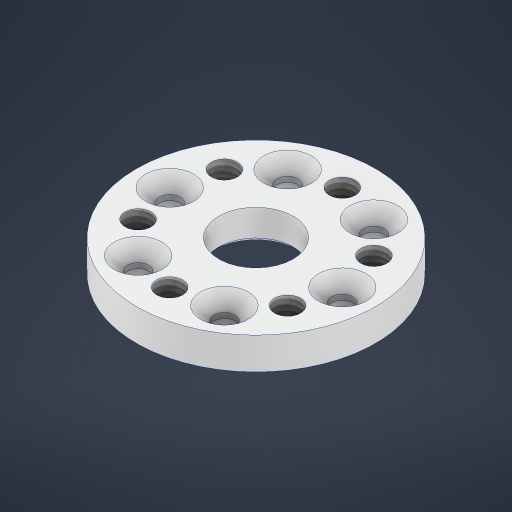
# Autodesk Inventor part: Carier_Plate_GB
Saved by Autodesk Inventor 2024.2 (Build 282272000, 272)
## iProperties
Created: 2026-01-04
Part Number: Carier_Plate_GB
Material: Aluminum 6061
Document SubType Name: Modeling
Designer: 4aida
Density: 2.7 g/cm^3
Appearance: Aluminum - Flat
Author: 4aida
Autodesk Inventor part; units mm, degrees
ref_plane "YZ Plane" through (0, 0, 0) normal (1, 0, 0) x (0, 1, 0)
ref_plane "XZ Plane" through (0, 0, 0) normal (0, 1, 0) x (-1, 0, 0)
ref_plane "XY Plane" through (0, 0, 0) normal (0, 0, 1) x (1, 0, 0)
sketch "Sketch1" plane through (0, 0, 0) normal (0, 1, 0) x (-1, 0, 0)
  circle A0 centre (0, 0) radius 22.5
  dimension "d0" = 45
  constraints: 1 centre point, 1 coincident
  measures "d0" diameter of A0
extrude "Extrusion1" add sketch "Sketch1" along normal mid plane 6
sketch "Sketch2" plane through (0, -3, 0) normal (0, -1, 0) x (1, 0, 0)
  point P0 (0, 0)
  point P1 (16.25, 0)
  dimension "d3" = 16.25
  constraints: 1 horizontal alignment
  measures "d3" distance of point (16.25, 0) point (0, 0)
hole "Hole1" at (16.25, -3, 0) direction (0, 1, 0) diameter 4 depth 6 counterbore diameter 6 counterbore depth 2.5
chamfer "Chamfer1" distance 2.5 angle 45 1 edges at (16.25, 3, 2)
pattern_circular "Circular Pattern1" count 6 over 360 about axis through (0, 0, 0) along (0, 1, 0) of "Hole1", "Chamfer1"
sketch "Sketch3" plane through (0, 3, 0) normal (0, 1, 0) x (1, 0, 0)
  point P0 (0, 0)
  point P1 (0, -16.25)
  dimension "d17" = 16.25
  constraints: 1 vertical alignment
  measures "d17" distance of point (0, 0) point (0, -16.25)
hole "Hole2" at (0, 3, 16.25) direction (0, -1, 0) diameter 4.917 depth 6 thread size "M6x1" class "6H" standard "ANSI Metric M Profile"
pattern_circular "Circular Pattern2" count 6 over 360 about axis through (0, 0, 0) along (0, 1, 0) of "Hole2"
sketch "Sketch5" plane through (0, -3, 0) normal (0, -1, 0) x (1, 0, 0)
  point P0 (0, 0)
  point P1 (0, 0)
  constraints: 1 coincident
hole "Hole4" at (0, -3, 0) direction (0, 1, 0) diameter 14 depth 6 counterbore diameter 16 counterbore depth 1
body "Solid1"
